Autodesk Fusion 360 part; units mm, degrees
(part 2 of 2)
  arc A256 (140.0805, 189.4205) -> (138.5565, 190.9445) centre (138.5565, 189.4205) ccw
  line L301 (171.8305, 189.4205) -> (171.8305, 175.0695)
  line L302 (171.8305, 251.2695) -> (171.8305, 236.9185)
  arc A257 (173.3545, 190.9445) -> (171.8305, 189.4205) centre (173.3545, 189.4205) ccw
  arc A258 (162.3055, 165.5445) -> (171.8305, 175.0695) centre (162.3055, 175.0695) ccw
  line L303 (133.7305, 244.9195) -> (133.7305, 236.9185)
  arc A259 (171.8305, 236.9185) -> (173.3545, 235.3945) centre (173.3545, 236.9185) ccw
  arc A260 (413.1305, 189.4205) -> (411.6065, 190.9445) centre (411.6065, 189.4205) ccw
  line L304 (140.0805, 236.9185) -> (140.0805, 251.2695)
  line L305 (444.8805, 251.2695) -> (444.8805, 236.9185)
  arc A261 (449.7065, 235.3945) -> (451.2305, 236.9185) centre (449.7065, 236.9185) ccw
  circle A262 centre (155.9555, 251.2695) radius 4.3815
  arc A263 (149.6055, 260.7945) -> (140.0805, 251.2695) centre (149.6055, 251.2695) ccw
  arc A264 (630.5545, 190.9445) -> (629.0305, 189.4205) centre (630.5545, 189.4205) ccw
  line L306 (140.0805, 175.0695) -> (140.0805, 189.4205)
  line L307 (422.6555, 260.7945) -> (435.3555, 260.7945)
  arc A265 (171.8305, 251.2695) -> (162.3055, 260.7945) centre (162.3055, 251.2695) ccw
  line L308 (138.5565, 190.9445) -> (135.2545, 190.9445)
  line L309 (44.8305, 181.4195) -> (44.8305, 244.9195)
  line L310 (444.8805, 189.4205) -> (444.8805, 175.0695)
  arc A266 (444.8805, 251.2695) -> (435.3555, 260.7945) centre (435.3555, 251.2695) ccw
  line L311 (449.7065, 190.9445) -> (446.4045, 190.9445)
  arc A267 (444.8805, 236.9185) -> (446.4045, 235.3945) centre (446.4045, 236.9185) ccw
  line L312 (902.0805, 189.4205) -> (902.0805, 181.4195)
  line L313 (667.1305, 251.2695) -> (667.1305, 236.9185)
  line L314 (940.1805, 189.4205) -> (940.1805, 175.0695)
  line L315 (908.4305, 236.9185) -> (908.4305, 251.2695)
  arc A268 (902.0805, 236.9185) -> (903.6045, 235.3945) centre (903.6045, 236.9185) ccw
  arc A269 (629.0305, 236.9185) -> (630.5545, 235.3945) centre (630.5545, 236.9185) ccw
  line L316 (908.4305, 175.0695) -> (908.4305, 189.4205)
  line L317 (406.7805, 181.4195) -> (178.1805, 181.4195)
  arc A270 (411.6065, 235.3945) -> (413.1305, 236.9185) centre (411.6065, 236.9185) ccw
  line L318 (945.0065, 190.9445) -> (941.7045, 190.9445)
  line L319 (451.2305, 181.4195) -> (451.2305, 189.4205)
  line L320 (44.8305, 244.9195) -> (133.7305, 244.9195)
  line L321 (903.6045, 235.3945) -> (906.9065, 235.3945)
  line L322 (946.5305, 236.9185) -> (946.5305, 244.9195)
  line L323 (133.7305, 181.4195) -> (44.8305, 181.4195)
  line L324 (902.0805, 244.9195) -> (902.0805, 236.9185)
  circle A271 centre (2410.2055, 251.2695) radius 4.3815
  arc A272 (903.6045, 190.9445) -> (902.0805, 189.4205) centre (903.6045, 189.4205) ccw
  line L325 (906.9065, 190.9445) -> (903.6045, 190.9445)
  line L326 (940.1805, 251.2695) -> (940.1805, 236.9185)
  line L327 (1140.2055, 260.7945) -> (1152.9055, 260.7945)
  arc A273 (940.1805, 251.2695) -> (930.6555, 260.7945) centre (930.6555, 251.2695) ccw
  line L328 (1152.9055, 165.5445) -> (1140.2055, 165.5445)
  line L329 (2432.4305, 236.9185) -> (2432.4305, 244.9195)
  line L330 (941.7045, 235.3945) -> (945.0065, 235.3945)
  arc A274 (917.9555, 260.7945) -> (908.4305, 251.2695) centre (917.9555, 251.2695) ccw
  line L331 (435.3555, 165.5445) -> (422.6555, 165.5445)
  arc A275 (945.0065, 235.3945) -> (946.5305, 236.9185) centre (945.0065, 236.9185) ccw
  arc A276 (930.6555, 165.5445) -> (940.1805, 175.0695) centre (930.6555, 175.0695) ccw
  line L332 (2403.8555, 260.7945) -> (2416.5555, 260.7945)
  arc A277 (941.7045, 190.9445) -> (940.1805, 189.4205) centre (941.7045, 189.4205) ccw
  arc A278 (2394.3305, 175.0695) -> (2403.8555, 165.5445) centre (2403.8555, 175.0695) ccw
  arc A279 (908.4305, 175.0695) -> (917.9555, 165.5445) centre (917.9555, 175.0695) ccw
  arc A280 (908.4305, 189.4205) -> (906.9065, 190.9445) centre (906.9065, 189.4205) ccw
  line L333 (930.6555, 165.5445) -> (917.9555, 165.5445)
  arc A281 (133.7305, 236.9185) -> (135.2545, 235.3945) centre (135.2545, 236.9185) ccw
  line L334 (629.0305, 189.4205) -> (629.0305, 181.4195)
  line L335 (2432.4305, 181.4195) -> (2432.4305, 189.4205)
  line L336 (2426.0805, 251.2695) -> (2426.0805, 236.9185)
  arc A282 (435.3555, 165.5445) -> (444.8805, 175.0695) centre (435.3555, 175.0695) ccw
  line L337 (629.0305, 181.4195) -> (451.2305, 181.4195)
  line L338 (411.6065, 190.9445) -> (408.3045, 190.9445)
  line L339 (408.3045, 235.3945) -> (411.6065, 235.3945)
  arc A283 (135.2545, 190.9445) -> (133.7305, 189.4205) centre (135.2545, 189.4205) ccw
  arc A284 (178.1805, 189.4205) -> (176.6565, 190.9445) centre (176.6565, 189.4205) ccw
  arc A285 (406.7805, 236.9185) -> (408.3045, 235.3945) centre (408.3045, 236.9185) ccw
  line L340 (635.3805, 236.9185) -> (635.3805, 251.2695)
  line L341 (673.4805, 236.9185) -> (673.4805, 244.9195)
  arc A286 (940.1805, 236.9185) -> (941.7045, 235.3945) centre (941.7045, 236.9185) ccw
  arc A287 (413.1305, 175.0695) -> (422.6555, 165.5445) centre (422.6555, 175.0695) ccw
  line L342 (451.2305, 244.9195) -> (629.0305, 244.9195)
  arc A288 (946.5305, 189.4205) -> (945.0065, 190.9445) centre (945.0065, 189.4205) ccw
  line L343 (917.9555, 260.7945) -> (930.6555, 260.7945)
  line L344 (2521.3305, 244.9195) -> (2521.3305, 181.4195)
  arc A289 (906.9065, 235.3945) -> (908.4305, 236.9185) centre (906.9065, 236.9185) ccw
  circle A290 centre (924.3055, 175.0695) radius 4.3815
  line L345 (629.0305, 244.9195) -> (629.0305, 236.9185)
  circle A291 centre (924.3055, 251.2695) radius 4.3815
  line L346 (406.7805, 189.4205) -> (406.7805, 181.4195)
  line L347 (946.5305, 181.4195) -> (946.5305, 189.4205)
  arc A292 (408.3045, 190.9445) -> (406.7805, 189.4205) centre (408.3045, 189.4205) ccw
  arc A293 (451.2305, 189.4205) -> (449.7065, 190.9445) centre (449.7065, 189.4205) ccw
  circle A294 centre (429.0055, 251.2695) radius 4.3815
  arc A295 (1435.4805, 751.2685) -> (1437.0045, 749.7445) centre (1437.0045, 751.2685) ccw
  line L348 (1413.2555, 775.1445) -> (1425.9555, 775.1445)
  line L349 (1435.4805, 703.7705) -> (1435.4805, 689.4195)
  line L350 (1397.3805, 695.7695) -> (1168.7805, 695.7695)
  line L351 (1403.7305, 751.2685) -> (1403.7305, 765.6195)
  line L352 (1435.4805, 765.6195) -> (1435.4805, 751.2685)
  arc A296 (1635.5055, 775.1445) -> (1625.9805, 765.6195) centre (1635.5055, 765.6195) ccw
  line L353 (1621.1545, 749.7445) -> (1624.4565, 749.7445)
  arc A297 (1625.9805, 689.4195) -> (1635.5055, 679.8945) centre (1635.5055, 689.4195) ccw
  circle A298 centre (1641.8555, 765.6195) radius 4.3815
  arc A299 (1621.1545, 705.2945) -> (1619.6305, 703.7705) centre (1621.1545, 703.7705) ccw
  arc A300 (1624.4565, 749.7445) -> (1625.9805, 751.2685) centre (1624.4565, 751.2685) ccw
  arc A301 (1619.6305, 751.2685) -> (1621.1545, 749.7445) centre (1621.1545, 751.2685) ccw
  line L354 (1619.6305, 703.7705) -> (1619.6305, 695.7695)
  line L355 (1625.9805, 751.2685) -> (1625.9805, 765.6195)
  line L356 (1625.9805, 689.4195) -> (1625.9805, 703.7705)
  circle A302 centre (1641.8555, 689.4195) radius 4.3815
  line L357 (1937.1305, 695.7695) -> (1937.1305, 703.7705)
  arc A303 (1930.7805, 765.6195) -> (1921.2555, 775.1445) centre (1921.2555, 765.6195) ccw
  line L358 (1892.6805, 703.7705) -> (1892.6805, 695.7695)
  line L359 (1892.6805, 759.2695) -> (1892.6805, 751.2685)
  arc A304 (1894.2045, 705.2945) -> (1892.6805, 703.7705) centre (1894.2045, 703.7705) ccw
  line L360 (1932.3045, 749.7445) -> (1935.6065, 749.7445)
  line L361 (1664.0805, 759.2695) -> (1892.6805, 759.2695)
  arc A305 (1892.6805, 751.2685) -> (1894.2045, 749.7445) centre (1894.2045, 751.2685) ccw
  line L362 (1892.6805, 695.7695) -> (1664.0805, 695.7695)
  arc A306 (1403.7305, 703.7705) -> (1402.2065, 705.2945) centre (1402.2065, 703.7705) ccw
  arc A307 (1437.0045, 705.2945) -> (1435.4805, 703.7705) centre (1437.0045, 703.7705) ccw
  arc A308 (1398.9045, 705.2945) -> (1397.3805, 703.7705) centre (1398.9045, 703.7705) ccw
  arc A309 (1625.9805, 703.7705) -> (1624.4565, 705.2945) centre (1624.4565, 703.7705) ccw
  line L363 (1624.4565, 705.2945) -> (1621.1545, 705.2945)
  line L364 (1397.3805, 759.2695) -> (1397.3805, 751.2685)
  circle A310 centre (1419.6055, 689.4195) radius 4.3815
  arc A311 (1435.4805, 765.6195) -> (1425.9555, 775.1445) centre (1425.9555, 765.6195) ccw
  line L365 (1403.7305, 689.4195) -> (1403.7305, 703.7705)
  line L366 (1619.6305, 759.2695) -> (1619.6305, 751.2685)
  arc A312 (1403.7305, 689.4195) -> (1413.2555, 679.8945) centre (1413.2555, 689.4195) ccw
  line L367 (1921.2555, 679.8945) -> (1908.5555, 679.8945)
  arc A313 (1921.2555, 679.8945) -> (1930.7805, 689.4195) centre (1921.2555, 689.4195) ccw
  line L368 (1899.0305, 751.2685) -> (1899.0305, 765.6195)
  line L369 (1897.5065, 705.2945) -> (1894.2045, 705.2945)
  arc A314 (1937.1305, 703.7705) -> (1935.6065, 705.2945) centre (1935.6065, 703.7705) ccw
  line L370 (1935.6065, 705.2945) -> (1932.3045, 705.2945)
  line L371 (1908.5555, 775.1445) -> (1921.2555, 775.1445)
  arc A315 (1932.3045, 705.2945) -> (1930.7805, 703.7705) centre (1932.3045, 703.7705) ccw
  arc A316 (1899.0305, 703.7705) -> (1897.5065, 705.2945) centre (1897.5065, 703.7705) ccw
  line L372 (1930.7805, 703.7705) -> (1930.7805, 689.4195)
  line L373 (1930.7805, 765.6195) -> (1930.7805, 751.2685)
  line L374 (1168.7805, 759.2695) -> (1397.3805, 759.2695)
  circle A317 centre (1914.9055, 689.4195) radius 4.3815
  arc A318 (1908.5555, 775.1445) -> (1899.0305, 765.6195) centre (1908.5555, 765.6195) ccw
  arc A319 (1935.6065, 749.7445) -> (1937.1305, 751.2685) centre (1935.6065, 751.2685) ccw
  line L375 (1894.2045, 749.7445) -> (1897.5065, 749.7445)
  arc A320 (930.6555, 679.8945) -> (940.1805, 689.4195) centre (930.6555, 689.4195) ccw
  arc A321 (2394.3305, 689.4195) -> (2403.8555, 679.8945) centre (2403.8555, 689.4195) ccw
  arc A322 (2426.0805, 765.6195) -> (2416.5555, 775.1445) centre (2416.5555, 765.6195) ccw
  line L376 (1152.9055, 679.8945) -> (1140.2055, 679.8945)
  arc A323 (2432.4305, 703.7705) -> (2430.9065, 705.2945) centre (2430.9065, 703.7705) ccw
  arc A324 (1413.2555, 775.1445) -> (1403.7305, 765.6195) centre (1413.2555, 765.6195) ccw
  arc A325 (1397.3805, 751.2685) -> (1398.9045, 749.7445) centre (1398.9045, 751.2685) ccw
  line L377 (1425.9555, 679.8945) -> (1413.2555, 679.8945)
  circle A326 centre (1419.6055, 765.6195) radius 4.3815
  line L378 (1398.9045, 749.7445) -> (1402.2065, 749.7445)
  arc A327 (1402.2065, 749.7445) -> (1403.7305, 751.2685) centre (1402.2065, 751.2685) ccw
  line L379 (1397.3805, 703.7705) -> (1397.3805, 695.7695)
  line L380 (1937.1305, 751.2685) -> (1937.1305, 759.2695)
  arc A328 (2154.5545, 705.2945) -> (2153.0305, 703.7705) centre (2154.5545, 703.7705) ccw
  arc A329 (1162.4305, 751.2685) -> (1163.9545, 749.7445) centre (1163.9545, 751.2685) ccw
  arc A330 (1163.9545, 705.2945) -> (1162.4305, 703.7705) centre (1163.9545, 703.7705) ccw
  line L381 (1168.7805, 751.2685) -> (1168.7805, 759.2695)
  line L382 (1162.4305, 703.7705) -> (1162.4305, 689.4195)
  line L383 (633.8565, 705.2945) -> (630.5545, 705.2945)
  arc A331 (667.1305, 751.2685) -> (668.6545, 749.7445) centre (668.6545, 751.2685) ccw
  line L384 (635.3805, 689.4195) -> (635.3805, 703.7705)
  line L385 (941.7045, 749.7445) -> (945.0065, 749.7445)
  line L386 (1124.3305, 695.7695) -> (946.5305, 695.7695)
  line L387 (635.3805, 751.2685) -> (635.3805, 765.6195)
  arc A332 (668.6545, 705.2945) -> (667.1305, 703.7705) centre (668.6545, 703.7705) ccw
  circle A333 centre (651.2555, 689.4195) radius 4.3815
  line L388 (657.6055, 679.8945) -> (644.9055, 679.8945)
  arc A334 (667.1305, 765.6195) -> (657.6055, 775.1445) centre (657.6055, 765.6195) ccw
  line L389 (908.4305, 689.4195) -> (908.4305, 703.7705)
  arc A335 (673.4805, 703.7705) -> (671.9565, 705.2945) centre (671.9565, 703.7705) ccw
  arc A336 (671.9565, 749.7445) -> (673.4805, 751.2685) centre (671.9565, 751.2685) ccw
  arc A337 (908.4305, 689.4195) -> (917.9555, 679.8945) centre (917.9555, 689.4195) ccw
  line L390 (2387.9805, 759.2695) -> (2387.9805, 751.2685)
  line L391 (2387.9805, 695.7695) -> (2159.3805, 695.7695)
  arc A338 (2389.5045, 705.2945) -> (2387.9805, 703.7705) centre (2389.5045, 703.7705) ccw
  arc A339 (633.8565, 749.7445) -> (635.3805, 751.2685) centre (633.8565, 751.2685) ccw
  arc A340 (945.0065, 749.7445) -> (946.5305, 751.2685) centre (945.0065, 751.2685) ccw
  line L392 (946.5305, 759.2695) -> (1124.3305, 759.2695)
  line L393 (946.5305, 751.2685) -> (946.5305, 759.2695)
  line L394 (2432.4305, 759.2695) -> (2521.3305, 759.2695)
  line L395 (940.1805, 703.7705) -> (940.1805, 689.4195)
  line L396 (940.1805, 765.6195) -> (940.1805, 751.2685)
  line L397 (930.6555, 679.8945) -> (917.9555, 679.8945)
  line L398 (2387.9805, 703.7705) -> (2387.9805, 695.7695)
  line L399 (2521.3305, 695.7695) -> (2432.4305, 695.7695)
  line L400 (667.1305, 765.6195) -> (667.1305, 751.2685)
  line L401 (2521.3305, 759.2695) -> (2521.3305, 695.7695)
  line L402 (668.6545, 749.7445) -> (671.9565, 749.7445)
  line L403 (2159.3805, 759.2695) -> (2387.9805, 759.2695)
  arc A341 (2387.9805, 751.2685) -> (2389.5045, 749.7445) centre (2389.5045, 751.2685) ccw
  line L404 (902.0805, 759.2695) -> (902.0805, 751.2685)
  arc A342 (1168.7805, 703.7705) -> (1167.2565, 705.2945) centre (1167.2565, 703.7705) ccw
  arc A343 (1152.9055, 679.8945) -> (1162.4305, 689.4195) centre (1152.9055, 689.4195) ccw
  line L405 (1168.7805, 695.7695) -> (1168.7805, 703.7705)
  line L406 (1899.0305, 689.4195) -> (1899.0305, 703.7705)
  arc A344 (1930.7805, 751.2685) -> (1932.3045, 749.7445) centre (1932.3045, 751.2685) ccw
  circle A345 centre (1146.5555, 765.6195) radius 4.3815
  line L407 (2121.2805, 689.4195) -> (2121.2805, 703.7705)
  line L408 (1129.1565, 705.2945) -> (1125.8545, 705.2945)
  arc A346 (1124.3305, 751.2685) -> (1125.8545, 749.7445) centre (1125.8545, 751.2685) ccw
  arc A347 (2153.0305, 751.2685) -> (2154.5545, 749.7445) centre (2154.5545, 751.2685) ccw
  line L409 (2130.8055, 775.1445) -> (2143.5055, 775.1445)
  arc A348 (1130.6805, 689.4195) -> (1140.2055, 679.8945) centre (1140.2055, 689.4195) ccw
  line L410 (2114.9305, 759.2695) -> (2114.9305, 751.2685)
  line L411 (1130.6805, 689.4195) -> (1130.6805, 703.7705)
  line L412 (1125.8545, 749.7445) -> (1129.1565, 749.7445)
  line L413 (1124.3305, 703.7705) -> (1124.3305, 695.7695)
  line L414 (2159.3805, 695.7695) -> (2159.3805, 703.7705)
  arc A349 (2143.5055, 679.8945) -> (2153.0305, 689.4195) centre (2143.5055, 689.4195) ccw
  line L415 (1140.2055, 775.1445) -> (1152.9055, 775.1445)
  arc A350 (1659.2545, 705.2945) -> (1657.7305, 703.7705) centre (1659.2545, 703.7705) ccw
  line L416 (1657.7305, 765.6195) -> (1657.7305, 751.2685)
  line L417 (1664.0805, 695.7695) -> (1664.0805, 703.7705)
  arc A351 (1657.7305, 751.2685) -> (1659.2545, 749.7445) centre (1659.2545, 751.2685) ccw
  line L418 (1659.2545, 749.7445) -> (1662.5565, 749.7445)
  arc A352 (1899.0305, 689.4195) -> (1908.5555, 679.8945) centre (1908.5555, 689.4195) ccw
  arc A353 (1662.5565, 749.7445) -> (1664.0805, 751.2685) centre (1662.5565, 751.2685) ccw
  arc A354 (1664.0805, 703.7705) -> (1662.5565, 705.2945) centre (1662.5565, 703.7705) ccw
  line L419 (1664.0805, 751.2685) -> (1664.0805, 759.2695)
  arc A355 (1657.7305, 765.6195) -> (1648.2055, 775.1445) centre (1648.2055, 765.6195) ccw
  line L420 (1657.7305, 703.7705) -> (1657.7305, 689.4195)
  arc A356 (1648.2055, 679.8945) -> (1657.7305, 689.4195) centre (1648.2055, 689.4195) ccw
  line L421 (1662.5565, 705.2945) -> (1659.2545, 705.2945)
  arc A357 (1425.9555, 679.8945) -> (1435.4805, 689.4195) centre (1425.9555, 689.4195) ccw
  line L422 (1437.0045, 749.7445) -> (1440.3065, 749.7445)
  line L423 (1402.2065, 705.2945) -> (1398.9045, 705.2945)
  line L424 (1440.3065, 705.2945) -> (1437.0045, 705.2945)
  line L425 (2121.2805, 751.2685) -> (2121.2805, 765.6195)
  arc A358 (1129.1565, 749.7445) -> (1130.6805, 751.2685) centre (1129.1565, 751.2685) ccw
  arc A359 (1130.6805, 703.7705) -> (1129.1565, 705.2945) centre (1129.1565, 703.7705) ccw
  line L426 (2119.7565, 705.2945) -> (2116.4545, 705.2945)
  arc A360 (2114.9305, 751.2685) -> (2116.4545, 749.7445) centre (2116.4545, 751.2685) ccw
  arc A361 (1140.2055, 775.1445) -> (1130.6805, 765.6195) centre (1140.2055, 765.6195) ccw
  arc A362 (1125.8545, 705.2945) -> (1124.3305, 703.7705) centre (1125.8545, 703.7705) ccw
  arc A363 (2119.7565, 749.7445) -> (2121.2805, 751.2685) centre (2119.7565, 751.2685) ccw
  arc A364 (2116.4545, 705.2945) -> (2114.9305, 703.7705) centre (2116.4545, 703.7705) ccw
  arc A365 (2130.8055, 775.1445) -> (2121.2805, 765.6195) centre (2130.8055, 765.6195) ccw
  line L427 (2143.5055, 679.8945) -> (2130.8055, 679.8945)
  line L428 (2116.4545, 749.7445) -> (2119.7565, 749.7445)
  line L429 (1124.3305, 759.2695) -> (1124.3305, 751.2685)
  line L430 (2153.0305, 765.6195) -> (2153.0305, 751.2685)
  line L431 (2153.0305, 703.7705) -> (2153.0305, 689.4195)
  circle A366 centre (1146.5555, 689.4195) radius 4.3815
  arc A367 (2159.3805, 703.7705) -> (2157.8565, 705.2945) centre (2157.8565, 703.7705) ccw
  line L432 (2154.5545, 749.7445) -> (2157.8565, 749.7445)
  line L433 (1130.6805, 751.2685) -> (1130.6805, 765.6195)
  line L434 (140.0805, 689.4195) -> (140.0805, 703.7705)
  arc A368 (629.0305, 751.2685) -> (630.5545, 749.7445) centre (630.5545, 751.2685) ccw
  line L435 (629.0305, 759.2695) -> (629.0305, 751.2685)
  line L436 (449.7065, 705.2945) -> (446.4045, 705.2945)
  line L437 (435.3555, 679.8945) -> (422.6555, 679.8945)
  circle A369 centre (429.0055, 689.4195) radius 4.3815
  arc A370 (449.7065, 749.7445) -> (451.2305, 751.2685) centre (449.7065, 751.2685) ccw
  arc A371 (413.1305, 689.4195) -> (422.6555, 679.8945) centre (422.6555, 689.4195) ccw
  line L438 (171.8305, 703.7705) -> (171.8305, 689.4195)
  arc A372 (435.3555, 679.8945) -> (444.8805, 689.4195) centre (435.3555, 689.4195) ccw
  arc A373 (135.2545, 705.2945) -> (133.7305, 703.7705) centre (135.2545, 703.7705) ccw
  line L439 (133.7305, 759.2695) -> (133.7305, 751.2685)
  line L440 (451.2305, 759.2695) -> (629.0305, 759.2695)
  line L441 (451.2305, 695.7695) -> (451.2305, 703.7705)
  line L442 (446.4045, 749.7445) -> (449.7065, 749.7445)
  line L443 (133.7305, 695.7695) -> (44.8305, 695.7695)
  line L444 (44.8305, 759.2695) -> (133.7305, 759.2695)
  line L445 (413.1305, 751.2685) -> (413.1305, 765.6195)
  line L446 (140.0805, 751.2685) -> (140.0805, 765.6195)
  circle A374 centre (155.9555, 765.6195) radius 4.3815
  line L447 (178.1805, 759.2695) -> (406.7805, 759.2695)
  line L448 (444.8805, 765.6195) -> (444.8805, 751.2685)
  arc A375 (451.2305, 703.7705) -> (449.7065, 705.2945) centre (449.7065, 703.7705) ccw
  line L449 (135.2545, 749.7445) -> (138.5565, 749.7445)
  arc A376 (413.1305, 703.7705) -> (411.6065, 705.2945) centre (411.6065, 703.7705) ccw
  line L450 (408.3045, 749.7445) -> (411.6065, 749.7445)
  circle A377 centre (155.9555, 689.4195) radius 4.3815
  arc A378 (162.3055, 679.8945) -> (171.8305, 689.4195) centre (162.3055, 689.4195) ccw
  circle A379 centre (429.0055, 765.6195) radius 4.3815
  line L451 (406.7805, 759.2695) -> (406.7805, 751.2685)
  arc A380 (444.8805, 751.2685) -> (446.4045, 749.7445) centre (446.4045, 751.2685) ccw
  line L452 (178.1805, 751.2685) -> (178.1805, 759.2695)
  line L453 (413.1305, 689.4195) -> (413.1305, 703.7705)
  arc A381 (422.6555, 775.1445) -> (413.1305, 765.6195) centre (422.6555, 765.6195) ccw
  arc A382 (444.8805, 765.6195) -> (435.3555, 775.1445) centre (435.3555, 765.6195) ccw
  line L454 (44.8305, 695.7695) -> (44.8305, 759.2695)
  arc A383 (138.5565, 749.7445) -> (140.0805, 751.2685) centre (138.5565, 751.2685) ccw
  arc A384 (630.5545, 705.2945) -> (629.0305, 703.7705) centre (630.5545, 703.7705) ccw
  arc A385 (149.6055, 775.1445) -> (140.0805, 765.6195) centre (149.6055, 765.6195) ccw
  line L455 (173.3545, 749.7445) -> (176.6565, 749.7445)
  line L456 (133.7305, 703.7705) -> (133.7305, 695.7695)
  line L457 (629.0305, 703.7705) -> (629.0305, 695.7695)
  line L458 (178.1805, 695.7695) -> (178.1805, 703.7705)
  line L459 (451.2305, 751.2685) -> (451.2305, 759.2695)
  arc A386 (411.6065, 749.7445) -> (413.1305, 751.2685) centre (411.6065, 751.2685) ccw
  line L460 (411.6065, 705.2945) -> (408.3045, 705.2945)
  line L461 (444.8805, 703.7705) -> (444.8805, 689.4195)
  line L462 (629.0305, 695.7695) -> (451.2305, 695.7695)
  line L463 (176.6565, 705.2945) -> (173.3545, 705.2945)
  line L464 (422.6555, 775.1445) -> (435.3555, 775.1445)
  arc A387 (446.4045, 705.2945) -> (444.8805, 703.7705) centre (446.4045, 703.7705) ccw
  circle A388 centre (2410.2055, 765.6195) radius 4.3815
  line L465 (673.4805, 759.2695) -> (902.0805, 759.2695)
  line L466 (2394.3305, 751.2685) -> (2394.3305, 765.6195)
  line L467 (2403.8555, 775.1445) -> (2416.5555, 775.1445)
  arc A389 (906.9065, 749.7445) -> (908.4305, 751.2685) centre (906.9065, 751.2685) ccw
  line L468 (2430.9065, 705.2945) -> (2427.6045, 705.2945)
  line L469 (902.0805, 695.7695) -> (673.4805, 695.7695)
  line L470 (908.4305, 751.2685) -> (908.4305, 765.6195)
  circle A390 centre (924.3055, 689.4195) radius 4.3815
  line L471 (917.9555, 775.1445) -> (930.6555, 775.1445)
  line L472 (2389.5045, 749.7445) -> (2392.8065, 749.7445)
  arc A391 (2427.6045, 705.2945) -> (2426.0805, 703.7705) centre (2427.6045, 703.7705) ccw
  arc A392 (917.9555, 775.1445) -> (908.4305, 765.6195) centre (917.9555, 765.6195) ccw
  arc A393 (2430.9065, 749.7445) -> (2432.4305, 751.2685) centre (2430.9065, 751.2685) ccw
  line L473 (2432.4305, 695.7695) -> (2432.4305, 703.7705)
  arc A394 (946.5305, 703.7705) -> (945.0065, 705.2945) centre (945.0065, 703.7705) ccw
  line L474 (902.0805, 703.7705) -> (902.0805, 695.7695)
  line L475 (2416.5555, 679.8945) -> (2403.8555, 679.8945)
  line L476 (903.6045, 749.7445) -> (906.9065, 749.7445)
  line L477 (945.0065, 705.2945) -> (941.7045, 705.2945)
  line L478 (1937.1305, 759.2695) -> (2114.9305, 759.2695)
  arc A395 (903.6045, 705.2945) -> (902.0805, 703.7705) centre (903.6045, 703.7705) ccw
  line L479 (2427.6045, 749.7445) -> (2430.9065, 749.7445)
  line L480 (946.5305, 695.7695) -> (946.5305, 703.7705)
  circle A396 centre (924.3055, 765.6195) radius 4.3815
  line L481 (906.9065, 705.2945) -> (903.6045, 705.2945)
  arc A397 (940.1805, 765.6195) -> (930.6555, 775.1445) centre (930.6555, 765.6195) ccw
  arc A398 (2392.8065, 749.7445) -> (2394.3305, 751.2685) centre (2392.8065, 751.2685) ccw
  circle A399 centre (2410.2055, 689.4195) radius 4.3815
  line L482 (2114.9305, 695.7695) -> (1937.1305, 695.7695)
  arc A400 (902.0805, 751.2685) -> (903.6045, 749.7445) centre (903.6045, 751.2685) ccw
  arc A401 (2394.3305, 703.7705) -> (2392.8065, 705.2945) centre (2392.8065, 703.7705) ccw
  arc A402 (908.4305, 703.7705) -> (906.9065, 705.2945) centre (906.9065, 703.7705) ccw
  line L483 (2426.0805, 765.6195) -> (2426.0805, 751.2685)
  line L484 (2392.8065, 705.2945) -> (2389.5045, 705.2945)
  arc A403 (2416.5555, 679.8945) -> (2426.0805, 689.4195) centre (2416.5555, 689.4195) ccw
  arc A404 (941.7045, 705.2945) -> (940.1805, 703.7705) centre (941.7045, 703.7705) ccw
  arc A405 (2426.0805, 751.2685) -> (2427.6045, 749.7445) centre (2427.6045, 751.2685) ccw
  line L485 (2394.3305, 689.4195) -> (2394.3305, 703.7705)
  arc A406 (2403.8555, 775.1445) -> (2394.3305, 765.6195) centre (2403.8555, 765.6195) ccw
  line L486 (2426.0805, 703.7705) -> (2426.0805, 689.4195)
  arc A407 (940.1805, 751.2685) -> (941.7045, 749.7445) centre (941.7045, 751.2685) ccw
  line L487 (2432.4305, 751.2685) -> (2432.4305, 759.2695)
  line L488 (1163.9545, 749.7445) -> (1167.2565, 749.7445)
  circle A408 centre (2137.1555, 765.6195) radius 4.3815
  line L489 (2114.9305, 703.7705) -> (2114.9305, 695.7695)
  circle A409 centre (2137.1555, 689.4195) radius 4.3815
  arc A410 (1167.2565, 749.7445) -> (1168.7805, 751.2685) centre (1167.2565, 751.2685) ccw
  arc A411 (2157.8565, 749.7445) -> (2159.3805, 751.2685) centre (2157.8565, 751.2685) ccw
  line L490 (1167.2565, 705.2945) -> (1163.9545, 705.2945)
  line L491 (1162.4305, 765.6195) -> (1162.4305, 751.2685)
  arc A412 (1162.4305, 765.6195) -> (1152.9055, 775.1445) centre (1152.9055, 765.6195) ccw
  arc A413 (2121.2805, 689.4195) -> (2130.8055, 679.8945) centre (2130.8055, 689.4195) ccw
  line L492 (2159.3805, 751.2685) -> (2159.3805, 759.2695)
  line L493 (2157.8565, 705.2945) -> (2154.5545, 705.2945)
  arc A414 (2121.2805, 703.7705) -> (2119.7565, 705.2945) centre (2119.7565, 703.7705) ccw
  arc A415 (2153.0305, 765.6195) -> (2143.5055, 775.1445) centre (2143.5055, 765.6195) ccw
  circle A416 centre (651.2555, 765.6195) radius 4.3815
  arc A417 (635.3805, 703.7705) -> (633.8565, 705.2945) centre (633.8565, 703.7705) ccw
  line L494 (644.9055, 775.1445) -> (657.6055, 775.1445)
  line L495 (667.1305, 703.7705) -> (667.1305, 689.4195)
  line L496 (671.9565, 705.2945) -> (668.6545, 705.2945)
  line L497 (673.4805, 695.7695) -> (673.4805, 703.7705)
  line L498 (406.7805, 703.7705) -> (406.7805, 695.7695)
  line L499 (406.7805, 695.7695) -> (178.1805, 695.7695)
  arc A418 (406.7805, 751.2685) -> (408.3045, 749.7445) centre (408.3045, 751.2685) ccw
  line L500 (630.5545, 749.7445) -> (633.8565, 749.7445)
  line L501 (673.4805, 751.2685) -> (673.4805, 759.2695)
  arc A419 (657.6055, 679.8945) -> (667.1305, 689.4195) centre (657.6055, 689.4195) ccw
  arc A420 (635.3805, 689.4195) -> (644.9055, 679.8945) centre (644.9055, 689.4195) ccw
  arc A421 (408.3045, 705.2945) -> (406.7805, 703.7705) centre (408.3045, 703.7705) ccw
  arc A422 (644.9055, 775.1445) -> (635.3805, 765.6195) centre (644.9055, 765.6195) ccw
  circle A423 centre (1914.9055, 765.6195) radius 4.3815
  arc A424 (1897.5065, 749.7445) -> (1899.0305, 751.2685) centre (1897.5065, 751.2685) ccw
  line L502 (1648.2055, 679.8945) -> (1635.5055, 679.8945)
  line L503 (1635.5055, 775.1445) -> (1648.2055, 775.1445)
  line L504 (1441.8305, 695.7695) -> (1441.8305, 703.7705)
  line L505 (1441.8305, 751.2685) -> (1441.8305, 759.2695)
  line L506 (1619.6305, 695.7695) -> (1441.8305, 695.7695)
  arc A425 (1440.3065, 749.7445) -> (1441.8305, 751.2685) centre (1440.3065, 751.2685) ccw
  arc A426 (1441.8305, 703.7705) -> (1440.3065, 705.2945) centre (1440.3065, 703.7705) ccw
  line L507 (1441.8305, 759.2695) -> (1619.6305, 759.2695)
  arc A427 (171.8305, 765.6195) -> (162.3055, 775.1445) centre (162.3055, 765.6195) ccw
  line L508 (138.5565, 705.2945) -> (135.2545, 705.2945)
  arc A428 (176.6565, 749.7445) -> (178.1805, 751.2685) centre (176.6565, 751.2685) ccw
  arc A429 (178.1805, 703.7705) -> (176.6565, 705.2945) centre (176.6565, 703.7705) ccw
  arc A430 (173.3545, 705.2945) -> (171.8305, 703.7705) centre (173.3545, 703.7705) ccw
  line L509 (171.8305, 765.6195) -> (171.8305, 751.2685)
  arc A431 (140.0805, 689.4195) -> (149.6055, 679.8945) centre (149.6055, 689.4195) ccw
  arc A432 (133.7305, 751.2685) -> (135.2545, 749.7445) centre (135.2545, 751.2685) ccw
  line L510 (149.6055, 775.1445) -> (162.3055, 775.1445)
  arc A433 (171.8305, 751.2685) -> (173.3545, 749.7445) centre (173.3545, 751.2685) ccw
  arc A434 (140.0805, 703.7705) -> (138.5565, 705.2945) centre (138.5565, 703.7705) ccw
  line L511 (162.3055, 679.8945) -> (149.6055, 679.8945)
  arc A435 (1921.2555, 844.9945) -> (1930.7805, 854.5195) centre (1921.2555, 854.5195) ccw
  line L512 (1899.0305, 854.5195) -> (1899.0305, 868.8705)
  line L513 (1930.7805, 930.7195) -> (1930.7805, 916.3685)
  line L514 (1908.5555, 940.2445) -> (1921.2555, 940.2445)
  line L515 (1937.1305, 916.3685) -> (1937.1305, 924.3695)
  arc A436 (1397.3805, 916.3685) -> (1398.9045, 914.8445) centre (1398.9045, 916.3685) ccw
  arc A437 (1425.9555, 844.9945) -> (1435.4805, 854.5195) centre (1425.9555, 854.5195) ccw
  arc A438 (1403.7305, 854.5195) -> (1413.2555, 844.9945) centre (1413.2555, 854.5195) ccw
  line L516 (1440.3065, 870.3945) -> (1437.0045, 870.3945)
  line L517 (1403.7305, 916.3685) -> (1403.7305, 930.7195)
  circle A439 centre (1419.6055, 854.5195) radius 4.3815
  arc A440 (1398.9045, 870.3945) -> (1397.3805, 868.8705) centre (1398.9045, 868.8705) ccw
  arc A441 (1402.2065, 914.8445) -> (1403.7305, 916.3685) centre (1402.2065, 916.3685) ccw
  arc A442 (1413.2555, 940.2445) -> (1403.7305, 930.7195) centre (1413.2555, 930.7195) ccw
  arc A443 (1435.4805, 930.7195) -> (1425.9555, 940.2445) centre (1425.9555, 930.7195) ccw
  line L518 (1403.7305, 854.5195) -> (1403.7305, 868.8705)
  arc A444 (1435.4805, 916.3685) -> (1437.0045, 914.8445) centre (1437.0045, 916.3685) ccw
  line L519 (1413.2555, 940.2445) -> (1425.9555, 940.2445)
  arc A445 (1403.7305, 868.8705) -> (1402.2065, 870.3945) centre (1402.2065, 868.8705) ccw
  line L520 (1402.2065, 870.3945) -> (1398.9045, 870.3945)
  arc A446 (1437.0045, 870.3945) -> (1435.4805, 868.8705) centre (1437.0045, 868.8705) ccw
  line L521 (1425.9555, 844.9945) -> (1413.2555, 844.9945)
  line L522 (1435.4805, 868.8705) -> (1435.4805, 854.5195)
  line L523 (1899.0305, 916.3685) -> (1899.0305, 930.7195)
  arc A447 (1930.7805, 930.7195) -> (1921.2555, 940.2445) centre (1921.2555, 930.7195) ccw
  line L524 (1897.5065, 870.3945) -> (1894.2045, 870.3945)
  line L525 (1894.2045, 914.8445) -> (1897.5065, 914.8445)
  arc A448 (1899.0305, 854.5195) -> (1908.5555, 844.9945) centre (1908.5555, 854.5195) ccw
  arc A449 (1932.3045, 870.3945) -> (1930.7805, 868.8705) centre (1932.3045, 868.8705) ccw
  line L526 (1930.7805, 868.8705) -> (1930.7805, 854.5195)
  arc A450 (1659.2545, 870.3945) -> (1657.7305, 868.8705) centre (1659.2545, 868.8705) ccw
  line L527 (1664.0805, 860.8695) -> (1664.0805, 868.8705)
  arc A451 (1664.0805, 868.8705) -> (1662.5565, 870.3945) centre (1662.5565, 868.8705) ccw
  arc A452 (1657.7305, 930.7195) -> (1648.2055, 940.2445) centre (1648.2055, 930.7195) ccw
  line L528 (2121.2805, 916.3685) -> (2121.2805, 930.7195)
  line L529 (2116.4545, 914.8445) -> (2119.7565, 914.8445)
  line L530 (2159.3805, 916.3685) -> (2159.3805, 924.3695)
  line L531 (2153.0305, 868.8705) -> (2153.0305, 854.5195)
  line L532 (2130.8055, 940.2445) -> (2143.5055, 940.2445)
  line L533 (2159.3805, 860.8695) -> (2159.3805, 868.8705)
  line L534 (2121.2805, 854.5195) -> (2121.2805, 868.8705)
  arc A453 (2153.0305, 930.7195) -> (2143.5055, 940.2445) centre (2143.5055, 930.7195) ccw
  arc A454 (2157.8565, 914.8445) -> (2159.3805, 916.3685) centre (2157.8565, 916.3685) ccw
  line L535 (2157.8565, 870.3945) -> (2154.5545, 870.3945)
  arc A455 (2153.0305, 916.3685) -> (2154.5545, 914.8445) centre (2154.5545, 916.3685) ccw
  arc A456 (2114.9305, 916.3685) -> (2116.4545, 914.8445) centre (2116.4545, 916.3685) ccw
  arc A457 (2121.2805, 868.8705) -> (2119.7565, 870.3945) centre (2119.7565, 868.8705) ccw
  line L536 (2114.9305, 924.3695) -> (2114.9305, 916.3685)
  line L537 (2114.9305, 868.8705) -> (2114.9305, 860.8695)
  line L538 (1441.8305, 924.3695) -> (1619.6305, 924.3695)
  arc A458 (1440.3065, 914.8445) -> (1441.8305, 916.3685) centre (1440.3065, 916.3685) ccw
  line L539 (1397.3805, 868.8705) -> (1397.3805, 860.8695)
  line L540 (1397.3805, 924.3695) -> (1397.3805, 916.3685)
  arc A459 (1441.8305, 868.8705) -> (1440.3065, 870.3945) centre (1440.3065, 868.8705) ccw
  line L541 (1441.8305, 916.3685) -> (1441.8305, 924.3695)
  line L542 (1437.0045, 914.8445) -> (1440.3065, 914.8445)
  line L543 (1398.9045, 914.8445) -> (1402.2065, 914.8445)
  line L544 (1648.2055, 844.9945) -> (1635.5055, 844.9945)
  line L545 (1619.6305, 860.8695) -> (1441.8305, 860.8695)
  line L546 (1435.4805, 930.7195) -> (1435.4805, 916.3685)
  line L547 (1441.8305, 860.8695) -> (1441.8305, 868.8705)
  line L548 (1635.5055, 940.2445) -> (1648.2055, 940.2445)
  arc A460 (1899.0305, 868.8705) -> (1897.5065, 870.3945) centre (1897.5065, 868.8705) ccw
  circle A461 centre (1914.9055, 930.7195) radius 4.3815
  line L549 (1624.4565, 870.3945) -> (1621.1545, 870.3945)
  arc A462 (1625.9805, 854.5195) -> (1635.5055, 844.9945) centre (1635.5055, 854.5195) ccw
  circle A463 centre (1419.6055, 930.7195) radius 4.3815
  arc A464 (1930.7805, 916.3685) -> (1932.3045, 914.8445) centre (1932.3045, 916.3685) ccw
  line L550 (1935.6065, 870.3945) -> (1932.3045, 870.3945)
  arc A465 (1935.6065, 914.8445) -> (1937.1305, 916.3685) centre (1935.6065, 916.3685) ccw
  arc A466 (1897.5065, 914.8445) -> (1899.0305, 916.3685) centre (1897.5065, 916.3685) ccw
  arc A467 (1937.1305, 868.8705) -> (1935.6065, 870.3945) centre (1935.6065, 868.8705) ccw
  circle A468 centre (1914.9055, 854.5195) radius 4.3815
  line L551 (1921.2555, 844.9945) -> (1908.5555, 844.9945)
  arc A469 (1908.5555, 940.2445) -> (1899.0305, 930.7195) centre (1908.5555, 930.7195) ccw
  line L552 (1937.1305, 860.8695) -> (1937.1305, 868.8705)
  arc A470 (1621.1545, 870.3945) -> (1619.6305, 868.8705) centre (1621.1545, 868.8705) ccw
  circle A471 centre (1641.8555, 930.7195) radius 4.3815
  arc A472 (1635.5055, 940.2445) -> (1625.9805, 930.7195) centre (1635.5055, 930.7195) ccw
  line L553 (1619.6305, 868.8705) -> (1619.6305, 860.8695)
  arc A473 (1625.9805, 868.8705) -> (1624.4565, 870.3945) centre (1624.4565, 868.8705) ccw
  line L554 (1625.9805, 916.3685) -> (1625.9805, 930.7195)
  line L555 (1621.1545, 914.8445) -> (1624.4565, 914.8445)
  arc A474 (1624.4565, 914.8445) -> (1625.9805, 916.3685) centre (1624.4565, 916.3685) ccw
  arc A475 (1619.6305, 916.3685) -> (1621.1545, 914.8445) centre (1621.1545, 916.3685) ccw
  line L556 (2154.5545, 914.8445) -> (2157.8565, 914.8445)
  line L557 (2119.7565, 870.3945) -> (2116.4545, 870.3945)
  line L558 (2153.0305, 930.7195) -> (2153.0305, 916.3685)
  arc A476 (2154.5545, 870.3945) -> (2153.0305, 868.8705) centre (2154.5545, 868.8705) ccw
  arc A477 (2119.7565, 914.8445) -> (2121.2805, 916.3685) centre (2119.7565, 916.3685) ccw
  arc A478 (2116.4545, 870.3945) -> (2114.9305, 868.8705) centre (2116.4545, 868.8705) ccw
  arc A479 (2121.2805, 854.5195) -> (2130.8055, 844.9945) centre (2130.8055, 854.5195) ccw
  arc A480 (2159.3805, 868.8705) -> (2157.8565, 870.3945) centre (2157.8565, 868.8705) ccw
  circle A481 centre (2137.1555, 854.5195) radius 4.3815
  arc A482 (2143.5055, 844.9945) -> (2153.0305, 854.5195) centre (2143.5055, 854.5195) ccw
  line L559 (2143.5055, 844.9945) -> (2130.8055, 844.9945)
  circle A483 centre (2137.1555, 930.7195) radius 4.3815
  arc A484 (2130.8055, 940.2445) -> (2121.2805, 930.7195) centre (2130.8055, 930.7195) ccw
  arc A485 (449.7065, 914.8445) -> (451.2305, 916.3685) centre (449.7065, 916.3685) ccw
  line L560 (902.0805, 868.8705) -> (902.0805, 860.8695)
  arc A486 (444.8805, 916.3685) -> (446.4045, 914.8445) centre (446.4045, 916.3685) ccw
  line L561 (906.9065, 870.3945) -> (903.6045, 870.3945)
  line L562 (908.4305, 916.3685) -> (908.4305, 930.7195)
  arc A487 (444.8805, 930.7195) -> (435.3555, 940.2445) centre (435.3555, 930.7195) ccw
  arc A488 (411.6065, 914.8445) -> (413.1305, 916.3685) centre (411.6065, 916.3685) ccw
  line L563 (444.8805, 868.8705) -> (444.8805, 854.5195)
  arc A489 (171.8305, 930.7195) -> (162.3055, 940.2445) centre (162.3055, 930.7195) ccw
  arc A490 (940.1805, 930.7195) -> (930.6555, 940.2445) centre (930.6555, 930.7195) ccw
  arc A491 (902.0805, 916.3685) -> (903.6045, 914.8445) centre (903.6045, 916.3685) ccw
  circle A492 centre (429.0055, 930.7195) radius 4.3815
  line L564 (451.2305, 860.8695) -> (451.2305, 868.8705)
  arc A493 (140.0805, 854.5195) -> (149.6055, 844.9945) centre (149.6055, 854.5195) ccw
  line L565 (1662.5565, 870.3945) -> (1659.2545, 870.3945)
  arc A494 (1648.2055, 844.9945) -> (1657.7305, 854.5195) centre (1648.2055, 854.5195) ccw
  line L566 (1657.7305, 868.8705) -> (1657.7305, 854.5195)
  line L567 (1619.6305, 924.3695) -> (1619.6305, 916.3685)
  line L568 (1625.9805, 854.5195) -> (1625.9805, 868.8705)
  circle A495 centre (1641.8555, 854.5195) radius 4.3815
  line L569 (444.8805, 930.7195) -> (444.8805, 916.3685)
  line L570 (140.0805, 854.5195) -> (140.0805, 868.8705)
  line L571 (138.5565, 870.3945) -> (135.2545, 870.3945)
  arc A496 (908.4305, 868.8705) -> (906.9065, 870.3945) centre (906.9065, 868.8705) ccw
  line L572 (451.2305, 924.3695) -> (629.0305, 924.3695)
  arc A497 (903.6045, 870.3945) -> (902.0805, 868.8705) centre (903.6045, 868.8705) ccw
  line L573 (1124.3305, 860.8695) -> (946.5305, 860.8695)
  arc A498 (178.1805, 868.8705) -> (176.6565, 870.3945) centre (176.6565, 868.8705) ccw
  line L574 (940.1805, 930.7195) -> (940.1805, 916.3685)
  line L575 (941.7045, 914.8445) -> (945.0065, 914.8445)
  line L576 (930.6555, 844.9945) -> (917.9555, 844.9945)
  arc A499 (906.9065, 914.8445) -> (908.4305, 916.3685) centre (906.9065, 916.3685) ccw
  line L577 (413.1305, 916.3685) -> (413.1305, 930.7195)
  line L578 (449.7065, 870.3945) -> (446.4045, 870.3945)
  arc A500 (162.3055, 844.9945) -> (171.8305, 854.5195) centre (162.3055, 854.5195) ccw
  line L579 (629.0305, 868.8705) -> (629.0305, 860.8695)
  line L580 (422.6555, 940.2445) -> (435.3555, 940.2445)
  line L581 (171.8305, 930.7195) -> (171.8305, 916.3685)
  line L582 (411.6065, 870.3945) -> (408.3045, 870.3945)
  line L583 (451.2305, 916.3685) -> (451.2305, 924.3695)
  arc A501 (930.6555, 844.9945) -> (940.1805, 854.5195) centre (930.6555, 854.5195) ccw
  circle A502 centre (429.0055, 854.5195) radius 4.3815
  line L584 (44.8305, 860.8695) -> (44.8305, 924.3695)
  arc A503 (171.8305, 916.3685) -> (173.3545, 914.8445) centre (173.3545, 916.3685) ccw
  line L585 (946.5305, 860.8695) -> (946.5305, 868.8705)
  circle A504 centre (155.9555, 930.7195) radius 4.3815
  arc A505 (946.5305, 868.8705) -> (945.0065, 870.3945) centre (945.0065, 868.8705) ccw
  arc A506 (451.2305, 868.8705) -> (449.7065, 870.3945) centre (449.7065, 868.8705) ccw
  line L586 (903.6045, 914.8445) -> (906.9065, 914.8445)
  arc A507 (435.3555, 844.9945) -> (444.8805, 854.5195) centre (435.3555, 854.5195) ccw
  arc A508 (446.4045, 870.3945) -> (444.8805, 868.8705) centre (446.4045, 868.8705) ccw
  arc A509 (917.9555, 940.2445) -> (908.4305, 930.7195) centre (917.9555, 930.7195) ccw
  line L587 (435.3555, 844.9945) -> (422.6555, 844.9945)
  line L588 (413.1305, 854.5195) -> (413.1305, 868.8705)
  line L589 (635.3805, 916.3685) -> (635.3805, 930.7195)
  arc A510 (173.3545, 870.3945) -> (171.8305, 868.8705) centre (173.3545, 868.8705) ccw
  circle A511 centre (155.9555, 854.5195) radius 4.3815
  line L590 (902.0805, 924.3695) -> (902.0805, 916.3685)
  arc A512 (149.6055, 940.2445) -> (140.0805, 930.7195) centre (149.6055, 930.7195) ccw
  line L591 (162.3055, 844.9945) -> (149.6055, 844.9945)
  arc A513 (945.0065, 914.8445) -> (946.5305, 916.3685) centre (945.0065, 916.3685) ccw
  line L592 (176.6565, 870.3945) -> (173.3545, 870.3945)
  arc A514 (941.7045, 870.3945) -> (940.1805, 868.8705) centre (941.7045, 868.8705) ccw
  arc A515 (138.5565, 914.8445) -> (140.0805, 916.3685) centre (138.5565, 916.3685) ccw
  line L593 (668.6545, 914.8445) -> (671.9565, 914.8445)
  arc A516 (133.7305, 916.3685) -> (135.2545, 914.8445) centre (135.2545, 916.3685) ccw
  line L594 (133.7305, 860.8695) -> (44.8305, 860.8695)
  arc A517 (413.1305, 868.8705) -> (411.6065, 870.3945) centre (411.6065, 868.8705) ccw
  line L595 (178.1805, 860.8695) -> (178.1805, 868.8705)
  line L596 (946.5305, 924.3695) -> (1124.3305, 924.3695)
  arc A518 (629.0305, 916.3685) -> (630.5545, 914.8445) centre (630.5545, 916.3685) ccw
  line L597 (173.3545, 914.8445) -> (176.6565, 914.8445)
  line L598 (946.5305, 916.3685) -> (946.5305, 924.3695)
  arc A519 (140.0805, 868.8705) -> (138.5565, 870.3945) centre (138.5565, 868.8705) ccw
  line L599 (945.0065, 870.3945) -> (941.7045, 870.3945)
  circle A520 centre (924.3055, 930.7195) radius 4.3815
  arc A521 (413.1305, 854.5195) -> (422.6555, 844.9945) centre (422.6555, 854.5195) ccw
  arc A522 (422.6555, 940.2445) -> (413.1305, 930.7195) centre (422.6555, 930.7195) ccw
  arc A523 (940.1805, 916.3685) -> (941.7045, 914.8445) centre (941.7045, 916.3685) ccw
  line L600 (178.1805, 916.3685) -> (178.1805, 924.3695)
  line L601 (446.4045, 914.8445) -> (449.7065, 914.8445)
  line L602 (917.9555, 940.2445) -> (930.6555, 940.2445)
  line L603 (171.8305, 868.8705) -> (171.8305, 854.5195)
  line L604 (408.3045, 914.8445) -> (411.6065, 914.8445)
  line L605 (44.8305, 924.3695) -> (133.7305, 924.3695)
  line L606 (1124.3305, 924.3695) -> (1124.3305, 916.3685)
  arc A524 (671.9565, 914.8445) -> (673.4805, 916.3685) centre (671.9565, 916.3685) ccw
  line L607 (673.4805, 916.3685) -> (673.4805, 924.3695)
  arc A525 (635.3805, 854.5195) -> (644.9055, 844.9945) centre (644.9055, 854.5195) ccw
  arc A526 (668.6545, 870.3945) -> (667.1305, 868.8705) centre (668.6545, 868.8705) ccw
  line L608 (908.4305, 854.5195) -> (908.4305, 868.8705)
  line L609 (178.1805, 924.3695) -> (406.7805, 924.3695)
  arc A527 (408.3045, 870.3945) -> (406.7805, 868.8705) centre (408.3045, 868.8705) ccw
  circle A528 centre (1146.5555, 930.7195) radius 4.3815
  line L610 (629.0305, 860.8695) -> (451.2305, 860.8695)
  line L611 (133.7305, 924.3695) -> (133.7305, 916.3685)
  line L612 (1168.7805, 916.3685) -> (1168.7805, 924.3695)
  line L613 (406.7805, 868.8705) -> (406.7805, 860.8695)
  line L614 (406.7805, 924.3695) -> (406.7805, 916.3685)
  line L615 (940.1805, 868.8705) -> (940.1805, 854.5195)
  arc A529 (1168.7805, 868.8705) -> (1167.2565, 870.3945) centre (1167.2565, 868.8705) ccw
  circle A530 centre (1146.5555, 854.5195) radius 4.3815
  arc A531 (1130.6805, 868.8705) -> (1129.1565, 870.3945) centre (1129.1565, 868.8705) ccw
  arc A532 (1140.2055, 940.2445) -> (1130.6805, 930.7195) centre (1140.2055, 930.7195) ccw
  arc A533 (630.5545, 870.3945) -> (629.0305, 868.8705) centre (630.5545, 868.8705) ccw
  arc A534 (673.4805, 868.8705) -> (671.9565, 870.3945) centre (671.9565, 868.8705) ccw
  line L616 (1124.3305, 868.8705) -> (1124.3305, 860.8695)
  circle A535 centre (651.2555, 854.5195) radius 4.3815
  arc A536 (1130.6805, 854.5195) -> (1140.2055, 844.9945) centre (1140.2055, 854.5195) ccw
  arc A537 (644.9055, 940.2445) -> (635.3805, 930.7195) centre (644.9055, 930.7195) ccw
  line L617 (135.2545, 914.8445) -> (138.5565, 914.8445)
  arc A538 (635.3805, 868.8705) -> (633.8565, 870.3945) centre (633.8565, 868.8705) ccw
  line L618 (1129.1565, 870.3945) -> (1125.8545, 870.3945)
  line L619 (406.7805, 860.8695) -> (178.1805, 860.8695)
  line L620 (1125.8545, 914.8445) -> (1129.1565, 914.8445)
  line L621 (1167.2565, 870.3945) -> (1163.9545, 870.3945)
  line L622 (1163.9545, 914.8445) -> (1167.2565, 914.8445)
  line L623 (671.9565, 870.3945) -> (668.6545, 870.3945)
  circle A539 centre (924.3055, 854.5195) radius 4.3815
  line L624 (140.0805, 916.3685) -> (140.0805, 930.7195)
  arc A540 (667.1305, 916.3685) -> (668.6545, 914.8445) centre (668.6545, 916.3685) ccw
  line L625 (667.1305, 868.8705) -> (667.1305, 854.5195)
  arc A541 (908.4305, 854.5195) -> (917.9555, 844.9945) centre (917.9555, 854.5195) ccw
  line L626 (629.0305, 924.3695) -> (629.0305, 916.3685)
  line L627 (673.4805, 860.8695) -> (673.4805, 868.8705)
  line L628 (1130.6805, 916.3685) -> (1130.6805, 930.7195)
  line L629 (633.8565, 870.3945) -> (630.5545, 870.3945)
  line L630 (1162.4305, 930.7195) -> (1162.4305, 916.3685)
  line L631 (1130.6805, 854.5195) -> (1130.6805, 868.8705)
  line L632 (657.6055, 844.9945) -> (644.9055, 844.9945)
  line L633 (635.3805, 854.5195) -> (635.3805, 868.8705)
  arc A542 (176.6565, 914.8445) -> (178.1805, 916.3685) centre (176.6565, 916.3685) ccw
  arc A543 (1152.9055, 844.9945) -> (1162.4305, 854.5195) centre (1152.9055, 854.5195) ccw
  circle A544 centre (651.2555, 930.7195) radius 4.3815
  line L634 (667.1305, 930.7195) -> (667.1305, 916.3685)
  arc A545 (657.6055, 844.9945) -> (667.1305, 854.5195) centre (657.6055, 854.5195) ccw
  line L635 (133.7305, 868.8705) -> (133.7305, 860.8695)
  line L636 (630.5545, 914.8445) -> (633.8565, 914.8445)
  arc A546 (1129.1565, 914.8445) -> (1130.6805, 916.3685) centre (1129.1565, 916.3685) ccw
  line L637 (1140.2055, 940.2445) -> (1152.9055, 940.2445)
  arc A547 (135.2545, 870.3945) -> (133.7305, 868.8705) centre (135.2545, 868.8705) ccw
  line L638 (149.6055, 940.2445) -> (162.3055, 940.2445)
  line L639 (1152.9055, 844.9945) -> (1140.2055, 844.9945)
  line L640 (1168.7805, 860.8695) -> (1168.7805, 868.8705)
  arc A548 (1167.2565, 914.8445) -> (1168.7805, 916.3685) centre (1167.2565, 916.3685) ccw
  arc A549 (1662.5565, 914.8445) -> (1664.0805, 916.3685) centre (1662.5565, 916.3685) ccw
  line L641 (1659.2545, 914.8445) -> (1662.5565, 914.8445)
  line L642 (1657.7305, 930.7195) -> (1657.7305, 916.3685)
  arc A550 (1657.7305, 916.3685) -> (1659.2545, 914.8445) centre (1659.2545, 916.3685) ccw
  line L643 (1664.0805, 916.3685) -> (1664.0805, 924.3695)
  line L644 (1892.6805, 860.8695) -> (1664.0805, 860.8695)
  line L645 (1932.3045, 914.8445) -> (1935.6065, 914.8445)
  line L646 (1664.0805, 924.3695) -> (1892.6805, 924.3695)
  arc A551 (1892.6805, 916.3685) -> (1894.2045, 914.8445) centre (1894.2045, 916.3685) ccw
  line L647 (1892.6805, 868.8705) -> (1892.6805, 860.8695)
  arc A552 (1894.2045, 870.3945) -> (1892.6805, 868.8705) centre (1894.2045, 868.8705) ccw
  line L648 (1892.6805, 924.3695) -> (1892.6805, 916.3685)
  arc A553 (2427.6045, 870.3945) -> (2426.0805, 868.8705) centre (2427.6045, 868.8705) ccw
  arc A554 (2394.3305, 868.8705) -> (2392.8065, 870.3945) centre (2392.8065, 868.8705) ccw
  arc A555 (2416.5555, 844.9945) -> (2426.0805, 854.5195) centre (2416.5555, 854.5195) ccw
  arc A556 (2403.8555, 940.2445) -> (2394.3305, 930.7195) centre (2403.8555, 930.7195) ccw
  line L649 (2432.4305, 916.3685) -> (2432.4305, 924.3695)
  line L650 (2394.3305, 854.5195) -> (2394.3305, 868.8705)
  line L651 (2430.9065, 870.3945) -> (2427.6045, 870.3945)
  line L652 (2389.5045, 914.8445) -> (2392.8065, 914.8445)
  line L653 (2394.3305, 916.3685) -> (2394.3305, 930.7195)
  arc A557 (2426.0805, 930.7195) -> (2416.5555, 940.2445) centre (2416.5555, 930.7195) ccw
  arc A558 (2432.4305, 868.8705) -> (2430.9065, 870.3945) centre (2430.9065, 868.8705) ccw
  line L654 (2426.0805, 868.8705) -> (2426.0805, 854.5195)
  arc A559 (2392.8065, 914.8445) -> (2394.3305, 916.3685) centre (2392.8065, 916.3685) ccw
  arc A560 (2394.3305, 854.5195) -> (2403.8555, 844.9945) centre (2403.8555, 854.5195) ccw
  line L655 (1397.3805, 860.8695) -> (1168.7805, 860.8695)
  arc A561 (1124.3305, 916.3685) -> (1125.8545, 914.8445) centre (1125.8545, 916.3685) ccw
  line L656 (2392.8065, 870.3945) -> (2389.5045, 870.3945)
  line L657 (2114.9305, 860.8695) -> (1937.1305, 860.8695)
  arc A562 (667.1305, 930.7195) -> (657.6055, 940.2445) centre (657.6055, 930.7195) ccw
  line L658 (2432.4305, 860.8695) -> (2432.4305, 868.8705)
  arc A563 (2389.5045, 870.3945) -> (2387.9805, 868.8705) centre (2389.5045, 868.8705) ccw
  arc A564 (1125.8545, 870.3945) -> (1124.3305, 868.8705) centre (1125.8545, 868.8705) ccw
  arc A565 (2387.9805, 916.3685) -> (2389.5045, 914.8445) centre (2389.5045, 916.3685) ccw
  line L659 (2387.9805, 860.8695) -> (2159.3805, 860.8695)
  arc A566 (1162.4305, 916.3685) -> (1163.9545, 914.8445) centre (1163.9545, 916.3685) ccw
  line L660 (2416.5555, 844.9945) -> (2403.8555, 844.9945)
  arc A567 (406.7805, 916.3685) -> (408.3045, 914.8445) centre (408.3045, 916.3685) ccw
  arc A568 (633.8565, 914.8445) -> (635.3805, 916.3685) centre (633.8565, 916.3685) ccw
  arc A569 (1162.4305, 930.7195) -> (1152.9055, 940.2445) centre (1152.9055, 930.7195) ccw
  line L661 (1162.4305, 868.8705) -> (1162.4305, 854.5195)
  line L662 (644.9055, 940.2445) -> (657.6055, 940.2445)
  line L663 (2427.6045, 914.8445) -> (2430.9065, 914.8445)
  circle A570 centre (2410.2055, 854.5195) radius 4.3815
  line L664 (2426.0805, 930.7195) -> (2426.0805, 916.3685)
  line L665 (2387.9805, 924.3695) -> (2387.9805, 916.3685)
  line L666 (2432.4305, 924.3695) -> (2521.3305, 924.3695)
  arc A571 (2430.9065, 914.8445) -> (2432.4305, 916.3685) centre (2430.9065, 916.3685) ccw
  line L667 (2521.3305, 924.3695) -> (2521.3305, 860.8695)
  line L668 (2159.3805, 924.3695) -> (2387.9805, 924.3695)
  line L669 (1937.1305, 924.3695) -> (2114.9305, 924.3695)
  line L670 (2403.8555, 940.2445) -> (2416.5555, 940.2445)
  line L671 (902.0805, 860.8695) -> (673.4805, 860.8695)
  line L672 (2521.3305, 860.8695) -> (2432.4305, 860.8695)
  line L673 (1168.7805, 924.3695) -> (1397.3805, 924.3695)
  line L674 (673.4805, 924.3695) -> (902.0805, 924.3695)
  circle A572 centre (2410.2055, 930.7195) radius 4.3815
  line L675 (2387.9805, 868.8705) -> (2387.9805, 860.8695)
  arc A573 (2426.0805, 916.3685) -> (2427.6045, 914.8445) centre (2427.6045, 916.3685) ccw
  arc A574 (1163.9545, 870.3945) -> (1162.4305, 868.8705) centre (1163.9545, 868.8705) ccw
extrude "metal0" add sketch "metal0" against normal blind 31.75 makes body 1 at (704.9342, 1322.324, -10.5833) makes body 2 at (1695.5342, 1322.324, -10.5833) makes body 3 at (2190.8342, 1322.324, -10.5833) makes body 4 at (1200.2342, 1322.324, -10.5833) makes body 5 at (74.5319, 55.7318, 0) makes body 6 at (209.6342, 1322.324, -10.5833) makes body 7 at (74.5319, 220.8318, 0) makes body 8 at (2491.6291, 719.8572, 0) makes body 9 at (2491.6291, 884.9572, 0)
extrude "metal1" add sketch "metal1" against normal blind 63.5 from surface at -19.05 separate body makes body 10 at (2513.9932, 608.5262, -19.05) makes body 11 at (1028.0932, 608.5262, -19.05) makes body 12 at (1523.3932, 608.5262, -19.05) makes body 13 at (37.4932, 608.5262, -19.05) makes body 14 at (2018.6932, 608.5262, -19.05) makes body 15 at (532.7932, 608.5262, -19.05)
extrude "metal2" add sketch "metal2" against normal blind 76.2 from surface at -22.225 separate body makes body 16 at (791.709, 1385.824, -47.625) makes body 17 at (1774.0964, -144.018, -47.625)
